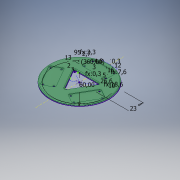
# Autodesk Inventor part: Stewart-Plate-inside
Saved by Autodesk Inventor 2018.2 (Build 222227000, 227)
## iProperties
Created: 2018-02-18
Part Number: Stewart-Plate-inside
Material: Generisch
Document SubType Name: Modeling
Designer: JochenAlt
Density: 1 g/cm^3
Appearance: Vorgabe
Author: JochenAlt
Autodesk Inventor part; units mm, degrees
ref_plane "YZ Plane" through (0, 0, 0) normal (1, 0, 0) x (0, 1, 0)
ref_plane "XZ Plane" through (0, 0, 0) normal (0, 1, 0) x (-1, 0, 0)
ref_plane "XY Plane" through (0, 0, 0) normal (0, 0, 1) x (1, 0, 0)
sketch "Skizze1" plane through (0, 0, 0) normal (0, 0, 1) x (1, 0, 0)
  line L0 (-11.2, 0) -> (11.2, 0) construction
  line L1 (-8, 36) -> (8, 36)
  line L2 (8, 36) -> (8, 33)
  line L3 (8, 33) -> (-8, 33)
  line L4 (-8, 33) -> (-8, 36)
  line L5 (1.5, 33) -> (-1.5, 33)
  line L6 (-1.5, 33) -> (-1.5, 28)
  line L7 (-1.5, 28) -> (1.5, 28)
  line L8 (1.5, 28) -> (1.5, 33)
  line L9 (0, 43.2) -> (0, -7.2) construction
  point P0 (0, 0)
  dimension "d10" = 3
  dimension "d14" = 16
  dimension "d23" = 5
  constraints: 16 end point, 4 parallel, 3 perpendicular, 2 horizontal, 2 point on line, 1 midpoint
  measures "d10" distance between parallel lines of L3 L1
  measures "d14" distance between parallel lines of L2 L4
  measures "d23" distance between parallel lines of L3 L7
extrude "Extrusion3" add sketch "Skizze1" against normal blind 7
fillet "Rundung1" radius 4 2 edges at (-8, 34.5, -7) (8, 34.5, -7)
sketch "Skizze2" plane through (-8, 36, 0) normal (0, 1, 0) x (1, 0, 0)
  circle A0 centre (3, 4) radius 1.1
  circle A1 centre (13, 4) radius 1.1
  line L0 (8, 0) -> (8, 7) construction
  line L1 (43, 0) -> (-27, 0) construction
  line L2 (-1.6221, 4) -> (19.0112, 4) construction
  line L3 (0, 7) -> (16, 7) construction
  line L4 (0, 0) -> (0, 7) projected
  point P0 (4, 7)
  point P1 (12, 7)
  point P2 (0, 3)
  dimension "d16" = 2.2
  dimension "d20" = 3
  dimension "d21" = 3
  constraints: 4 end point, 2 centre point, 1 equal radius, 1 horizontal, 1 midpoint, 1 point on line, 1 symmetric about line, 1 vertical
  measures "d16" diameter of A0
  measures "d20" distance between parallel lines of L3 L2
  measures "d21" distance from line of L4 A0.centre
extrude "Extrusion4" cut sketch "Skizze2" against normal up to next
chamfer "Fase1" distance 5 distance2 7 1 edges at (0, 28, -7) measured on face at (0, 28.5, -7)
pattern_circular "Runde Anordnung1" count 3 over 360 about axis through (0, 0, -10) along (0, 0, 1) of "Extrusion3", "Extrusion4", "Fase1", "Rundung1"
sketch "Skizze3" plane through (0, 0, 0) normal (0, 0, 1) x (1, 0, 0)
  line L0 (0, 71.493) -> (0, -71.493) construction
  circle A0 centre (0, 0) radius 39 construction
  circle A1 centre (0, 0) radius 47.5
  line L1 (18.5329, 12.7) -> (-18.5329, 12.7)
  line L2 (-20.265, 9.7) -> (-1.7321, -22.4)
  line L3 (20.265, 9.7) -> (1.7321, -22.4)
  line L4 (-14.1375, 8.1623) -> (10.9985, -6.35) construction
  line L5 (21.997, 12.7) -> (-10.9985, -6.35) construction
  line L6 (0.15, 49.6) -> (12.15, 49.6) construction
  line L7 (12.15, 49.6) -> (12.15, 23) construction
  line L8 (12.15, 23) -> (0.15, 23) construction
  line L9 (0.15, 23) -> (0.15, 49.6) construction
  line L10 (-0.15, 49.6) -> (-12.15, 49.6) construction
  line L11 (-12.15, 49.6) -> (-12.15, 23) construction
  line L12 (-12.15, 23) -> (-0.15, 23) construction
  line L13 (-0.15, 23) -> (-0.15, 49.6) construction
  line L14 (-17.45, 41.3) -> (17.45, 41.3)
  line L15 (19.75, 39) -> (19.75, 25)
  line L16 (17.45, 22.7) -> (-17.45, 22.7)
  line L17 (-19.75, 25) -> (-19.75, 39)
  arc A2 (-17.45, 41.3) -> (-19.75, 39) centre (-17.45, 39) ccw
  arc A3 (-19.75, 25) -> (-17.45, 22.7) centre (-17.45, 25) ccw
  arc A4 (17.45, 22.7) -> (19.75, 25) centre (17.45, 25) ccw
  arc A5 (19.75, 39) -> (17.45, 41.3) centre (17.45, 39) ccw
  circle A6 centre (-16.95, 38.65) radius 1.35
  circle A7 centre (-16.95, 25.65) radius 1.35
  circle A8 centre (16.95, 38.65) radius 1.35
  circle A9 centre (16.95, 25.65) radius 1.35
  line L18 (-19.75, 32.15) -> (19.75, 32.15) construction
  line L19 (-16.95, 38.65) -> (-16.95, 25.65) construction
  arc A10 (-27.0418, -35.7621) -> (-23.9, -36.604) centre (-25.05, -34.6121) ccw
  line L20 (-11.7756, -29.604) -> (-23.9, -36.604)
  circle A11 centre (-24.9969, -34.0041) radius 1.35
  line L21 (-27.0418, -35.7621) -> (-44.4918, -5.5379)
  circle A12 centre (-13.7386, -27.5041) radius 1.35
  arc A13 (-11.7756, -29.604) -> (-10.9338, -26.4621) centre (-12.9256, -27.6121) ccw
  line L22 (-28.3838, 3.7621) -> (-10.9338, -26.4621)
  arc A14 (-28.3838, 3.7621) -> (-31.5256, 4.604) centre (-30.3756, 2.6121) ccw
  circle A15 centre (-30.6886, 1.8541) radius 1.35
  arc A16 (-43.65, -2.396) -> (-44.4918, -5.5379) centre (-42.5, -4.3879) ccw
  circle A17 centre (-41.9469, -4.6459) radius 1.35
  line L23 (-43.65, -2.396) -> (-31.5256, 4.604)
  arc A18 (44.4918, -5.5379) -> (43.65, -2.396) centre (42.5, -4.3879) ccw
  line L24 (31.5256, 4.604) -> (43.65, -2.396)
  circle A19 centre (41.9469, -4.6459) radius 1.35
  line L25 (44.4918, -5.5379) -> (27.0418, -35.7621)
  circle A20 centre (30.6886, 1.8541) radius 1.35
  arc A21 (31.5256, 4.604) -> (28.3838, 3.7621) centre (30.3756, 2.6121) ccw
  line L26 (10.9338, -26.4621) -> (28.3838, 3.7621)
  arc A22 (10.9338, -26.4621) -> (11.7756, -29.604) centre (12.9256, -27.6121) ccw
  circle A23 centre (13.7386, -27.5041) radius 1.35
  arc A24 (23.9, -36.604) -> (27.0418, -35.7621) centre (25.05, -34.6121) ccw
  circle A25 centre (24.9969, -34.0041) radius 1.35
  line L27 (23.9, -36.604) -> (11.7756, -29.604)
  arc A26 (-18.5329, 12.7) -> (-20.265, 9.7) centre (-18.5329, 10.7) ccw
  arc A27 (-1.7321, -22.4) -> (1.7321, -22.4) centre (0, -21.4) ccw
  arc A28 (20.265, 9.7) -> (18.5329, 12.7) centre (18.5329, 10.7) ccw
  point P0 (-21.997, 12.7)
  point P1 (0, -25.4)
  point P2 (19.75, 12.7)
  point P3 (-14.2556, 12.7)
  point P4 (-13.3368, -2.3)
  point P5 (8.6603, -10.4)
  point P6 (-1.9919, -21.95)
  point P7 (-17.9677, -33.179)
  point P8 (-37.7177, 1.029)
  point P9 (37.7177, 1.029)
  point P10 (17.9677, -33.179)
  dimension "d140" = 60
  dimension "d146" = 0.3
  dimension "d147" = 26.6
  dimension "d148" = 12
  dimension "d150" = 0.3
  dimension "d151" = 18.6
  dimension "d152" = 2.3
  dimension "d153" = 13
  dimension "d154" = 7.6
  dimension "d155" = 4.8
  dimension "d158" = 360
  dimension "d160" = 10
  dimension "d161" = 2.7
  dimension "d164" = 23
  dimension "d184" = 2
  dimension "d189" = 95
  constraints: 54 end point, 30 point on circle, 28 centre point, 21 point on line, 14 tangent, 8 equal radius, 6 parallel, 4 perpendicular, 3 horizontal, 2 collinear, 2 midpoint, 2 symmetric about line, 1 coincident, 1 vertical, 97 other
  measures "d140" angle of L3 L1
  measures "d146" distance between parallel lines of L9 L13
  measures "d147" distance between parallel lines of L8 L6
  measures "d148" distance between parallel lines of L7 L9
  measures "d150" distance between parallel lines of L16 L8
  measures "d151" distance between parallel lines of L16 L14
  measures "d152" radius of A2
  measures "d153" distance of L19.end L19.start
  measures "d154" distance between parallel lines of L15 L7
  measures "d155" distance between parallel lines of L11 L19
  measures "d160" distance between parallel lines of L1 L16
  measures "d161" diameter of A6
  measures "d164" distance from line of point (0, 0) L8
  measures "d184" radius of A26
  measures "d189" diameter of A1
extrude "Extrusion11" add sketch "Skizze3" along normal blind 2.5 contours A1 | A28 L3 A27 L2 A26 L1 | L14 A5 L15 A4 L16 A3 L17 A2 | A6 | A7 | A8 | A9 | L21 A16 L23 A14 L22 A13 L20 A10 | A11 | A12 | A15 | A17 | L25 A24 L27 A22 L26 A21 L24 A18 | A19 | A20 | A23 | A25
extrude "Extrusion9" cut sketch "Skizze3" along normal blind 2.5 contours A28 L3 A27 L2 A26 L1 | L14 A5 L15 A4 L16 A3 L17 A2 | A6 | A7 | A8 | A9 | L21 A16 L23 A14 L22 A13 L20 A10 | A11 | A12 | A15 | A17 | L25 A24 L27 A22 L26 A21 L24 A18 | A19 | A20 | A23 | A25
extrude "Extrusion6" add sketch "Skizze3" along normal blind 1.5 contours L14 A5 L15 A4 L16 A3 L17 A2 | L21 A16 L23 A14 L22 A13 L20 A10 | L25 A24 L27 A22 L26 A21 L24 A18
fillet "Rundung4" radius 1 8 edges at (0, 12.7, 2.5) (10.9985, -6.35, 2.5) (-10.9985, -6.35, 2.5) (-10.9985, -6.35, 0) (10.9985, -6.35, 0) (0, 12.7, 0) (-47.5, 0, 2.5) (-47.5, 0, 0)
equation "\"d21\" = d20"
